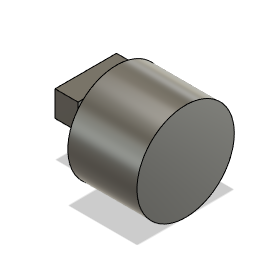
BottomTest v5 (Autodesk Fusion 360 archive; units mm, degrees)
design "StepperAndWheel"
Autodesk Fusion 360 part; units mm, degrees
sketch "草图1" plane through (0, 0, 0) normal (0, 1, 0) x (1, 0, 0)
  line L0 (0, -6) -> (9, -6)
  line L1 (9, -6) -> (9, 18)
  line L2 (9, 18) -> (0, 18)
  line L3 (0, 18) -> (0, -6)
  constraint horizontal L0
  constraint vertical L1
  constraint horizontal L2
  constraint vertical L3
extrude "拉伸1" add sketch "草图1" along normal blind 5 and the other way blind 0
extrude "拉伸2" add 1 faces at (3, 5, -10) along direction (0, 1, 0) blind 5
cylinder "圆柱体基本要素1" add diameter 3 height 9 placed x (0, 0, -1) y (0, 1, 0) z (1, 0, 0) at (9, 5, 0)
cylinder "圆柱体基本要素2" add diameter 38 height 27 placed x (0, 0, -1) y (0, 1, 0) z (1, 0, 0) at (18, 5, 0)
